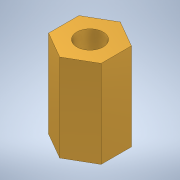
# Autodesk Inventor part: espaçador sext. 10mm
Saved by Autodesk Inventor 2021 (Build 250183000, 183)
## iProperties
Created: 2022-02-21
Part Number: espaçador sext. 10mm
Material: Generic
Document SubType Name: Modeling
Designer: Matheus
Density: 1 g/cm^3
Appearance: Default
Author: Matheus
Autodesk Inventor part; units mm, degrees
ref_plane "YZ Plane" through (0, 0, 0) normal (1, 0, 0) x (0, 1, 0)
ref_plane "XZ Plane" through (0, 0, 0) normal (0, 1, 0) x (-1, 0, 0)
ref_plane "XY Plane" through (0, 0, 0) normal (0, 0, 1) x (1, 0, 0)
sketch "Sketch1" plane through (0, 0, 0) normal (0, 1, 0) x (-1, 0, 0)
  circle A0 centre (0, 0) radius 1.5
  line L0 (-3, -1.7321) -> (-3, 1.7321)
  line L1 (-3, 1.7321) -> (0, 3.4641)
  line L2 (0, 3.4641) -> (3, 1.7321)
  line L3 (3, 1.7321) -> (3, -1.7321)
  line L4 (3, -1.7321) -> (0, -3.4641)
  line L5 (0, -3.4641) -> (-3, -1.7321)
  dimension "d0" = 3
  dimension "d1" = 6
  constraints: 12 end point, 2 coincident, 1 centre point, 1 vertical, 13 other
  measures "d0" diameter of A0
  measures "d1" distance between parallel lines of L3 L0
extrude "Extrusion1" add sketch "Sketch1" along normal blind 10
body "Solid1"
